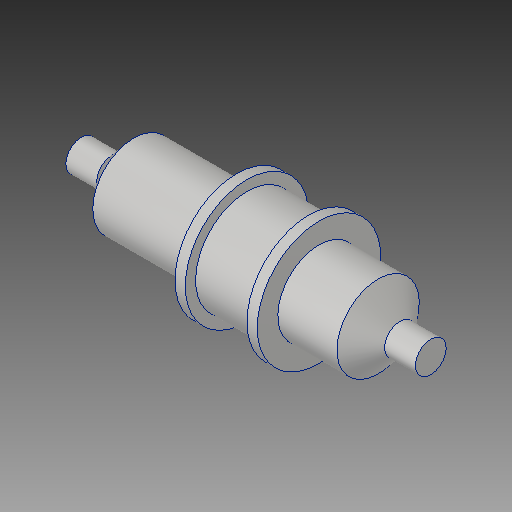
# Autodesk Inventor part: Axe de renvoie
Saved by Autodesk Inventor 2017 (Build 210142000, 142)
## iProperties
Company: FABLAB Frenchmakers
Part Number: Axe de renvoie
Material: Aluminium
Document SubType Name: Modeling
Designer: FABLAB Frenchmakers
Density: 2.7 g/cm^3
Appearance: Aluminium - Plat(2)
Mass: 4.42652 g
Surface Area: 10.3859 cm^2
Volume: 1.63945 cm^3
Stock Number: 1420-01-07
Project: 1420 Vauban 3D XL
Catalog Web Link: http://frenchmakers.com/
Autodesk Inventor part; units mm, degrees
ref_plane "YZ Plane" through (0, 0, 0) normal (1, 0, 0) x (0, 1, 0)
ref_plane "XZ Plane" through (0, 0, 0) normal (0, 1, 0) x (-1, 0, 0)
ref_plane "XY Plane" through (0, 0, 0) normal (0, 0, 1) x (1, 0, 0)
sketch "Esquisse1" plane through (0, 0, 0) normal (0, 0, 1) x (1, 0, 0)
  line L0 (-17, 0) -> (-17, 1.5)
  line L1 (-17, 1.5) -> (-14, 1.5)
  line L2 (-14, 1.5) -> (-11.875, 4)
  line L3 (-11.875, 4) -> (-1.875, 4)
  line L4 (-1.875, 4) -> (-1.875, 6)
  line L5 (-1.875, 6) -> (-0.875, 6)
  line L6 (-0.875, 6) -> (-0.875, 5)
  line L7 (5.125, 5) -> (5.125, 6)
  line L8 (5.125, 6) -> (6.125, 6)
  line L9 (6.125, 6) -> (6.125, 4)
  line L10 (6.125, 4) -> (11.875, 4)
  line L11 (11.875, 4) -> (14, 1.5)
  line L12 (14, 1.5) -> (17, 1.5)
  line L13 (17, 1.5) -> (17, 0)
  line L14 (-17, 0) -> (17, 0)
  line L15 (-44.329, 0) -> (0, 0)
  line L16 (-0.875, 5) -> (5.125, 5)
  dimension "d0" = 34
  dimension "d1" = 3
  dimension "d2" = 8
  dimension "d4" = 12
  dimension "d5" = 10
  dimension "d6" = 6
  dimension "d7" = 1
  dimension "d8" = 1
  dimension "d9" = 5.75
  dimension "d10" = 10
  dimension "d12" = 3
  dimension "d13" = 17
  dimension "d17" = 3
  constraints: 34 end point, 4 perpendicular, 4 point on line, 3 horizontal, 2 collinear, 1 coincident, 1 equal length, 1 vertical
  measures "d0" distance between parallel lines of L13 L0
  measures "d1" diameter of L12 L15
  measures "d2" diameter of L10 L15
  measures "d4" diameter of L8 L15
  measures "d5" diameter of L16 L15
  measures "d6" distance between parallel lines of L7 L6
  measures "d7" distance between parallel lines of L9 L7
  measures "d8" distance of L4.end L5.end
  measures "d9" distance of L9.end L10.end
  measures "d10" distance from line of L2.end L4
  measures "d12" distance of L11.end L12.end
  measures "d13" distance from line of point (0, 0) L0
  measures "d17" distance of L0.end L1.end
revolve "Révolution1" add sketch "Esquisse1" angle 360 about axis through (-44.329, 0, 0) along (1, 0, 0)
equation "\"d8\" = d7"
equation "\"d13\" = 0.5 * d0"
